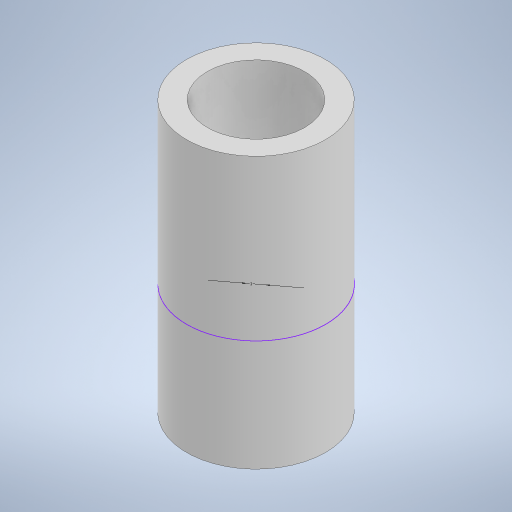
# Autodesk Inventor part: seegoals_adapter_puller_tool_v1
Saved by Autodesk Inventor 2024 (Build 280153000, 153)
## iProperties
Created: 2025-02-17
Part Number: seegoals_adapter_puller_tool_v1
Material: Generic
Document SubType Name: Modeling
Designer: Elev
Density: 1 g/cm^3
Appearance: Default
Author: Elev
Autodesk Inventor part; units mm, degrees
ref_plane "YZ Plane" through (0, 0, 0) normal (1, 0, 0) x (0, 1, 0)
ref_plane "XZ Plane" through (0, 0, 0) normal (0, 1, 0) x (-1, 0, 0)
ref_plane "XY Plane" through (0, 0, 0) normal (0, 0, 1) x (1, 0, 0)
sketch "Sketch1" plane through (0, 0, 0) normal (0, 1, 0) x (-1, 0, 0)
  line L0 (-1.7898, -3.1) -> (-3.5796, 0)
  line L1 (-3.5796, 0) -> (-1.7898, 3.1)
  line L2 (-1.7898, 3.1) -> (1.7898, 3.1)
  line L3 (1.7898, 3.1) -> (3.5796, 0)
  line L4 (3.5796, 0) -> (1.7898, -3.1)
  line L5 (1.7898, -3.1) -> (-1.7898, -3.1)
  circle A0 centre (0, 0) radius 5
  spline S0 degree 2 poles (1.7898, 3.1) (0, 2.8) (-1.7898, 3.1) knots 0 0 0 1 1 1
  spline S1 degree 2 poles (-1.7898, 3.1) (-2.4249, 1.4) (-3.5796, 0) knots 0 0 0 1 1 1
  spline S2 degree 2 poles (-3.5796, 0) (-2.4249, -1.4) (-1.7898, -3.1) knots 0 0 0 1 1 1
  spline S3 degree 2 poles (-1.7898, -3.1) (0, -2.8) (1.7898, -3.1) knots 0 0 0 1 1 1
  spline S4 degree 2 poles (1.7898, -3.1) (2.4249, -1.4) (3.5796, 0) knots 0 0 0 1 1 1
  spline S5 degree 2 poles (3.5796, 0) (2.4249, 1.4) (1.7898, 3.1) knots 0 0 0 1 1 1
  point P0 (0, 0)
  point P1 (0, 0)
  point P2 (0, -3.1)
  point P3 (0, 2.95)
  point P4 (0, 3.1)
  point P5 (-2.5548, 1.475)
  point P6 (-2.5548, -1.475)
  point P7 (0, -2.95)
  point P8 (2.5548, -1.475)
  point P9 (2.5548, 1.475)
  point P10 (1.7898, 3.1)
  point P11 (1.7898, 3.1)
  point P12 (1.7898, 3.1)
  dimension "d0" = 3.1
  dimension "d1" = 10
  dimension "d27" = 0.15
  dimension "d30" = 360
  constraints: 12 end point, 2 midpoint, 1 centre point, 1 coincident, 1 vertical alignment, 56 other
  measures "d0" distance from line of L5 point (0, 0)
  measures "d1" diameter of A0
  measures "d27" distance of point (0, 2.95) point (0, 3.1)
extrude "Extrusion1" add sketch "Sketch1" along normal blind 8 contours S3 L5 | L0 S2 | L1 S1 | S4 L4 | L2 S0 | S5 L3 | A0
sketch "Sketch2" plane through (0, 8, 0) normal (0, 1, 0) x (1, 0, 0)
  circle A0 centre (0, 0) radius 0.5
  circle A1 centre (0, 0) radius 5 projected
  circle A2 centre (0, 0) radius 5
  dimension "d4" = 1
  constraints: 2 centre point, 2 coincident
  measures "d4" diameter of A0
sketch "Sketch5" plane through (0, 0, 0) normal (0, 0, 1) x (1, 0, 0)
  line L0 (5, 8) -> (-5, 8) projected
  line L1 (5, 8) -> (5, 11.5)
  line L2 (5, 11.5) -> (3.5, 11.5)
  line L3 (5, 8) -> (0.5, 8)
  line L4 (0.5, 8) -> (3.5, 11.5)
  line L5 (0, 8) -> (0, 11)
  point P0 (0, 0)
  dimension "d20" = 3.5
  dimension "d21" = 1.5
  dimension "d22" = 4.5
  dimension "d23" = 3
  constraints: 10 end point, 2 vertical, 1 midpoint, 1 perpendicular, 1 point on line
  measures "d20" distance of L0.start L1.end
  measures "d21" distance of L1.end L2.end
  measures "d22" distance of L0.start L3.end
  measures "d23" distance of L5.start L5.end
revolve "Revolution1" add sketch "Sketch5" angle 360 about axis through (0, 8, 0) along (0, 1, 0)
sketch "Sketch7" plane through (0, 11.5, 0) normal (0, 1, 0) x (1, 0, 0)
  circle A0 centre (0, 0) radius 0.5 projected
  circle A1 centre (0, 0) radius 3.5
  circle A2 centre (0, 0) radius 5
  constraints: 2 centre point, 2 coincident
extrude "Extrusion2" add sketch "Sketch7" along normal blind 8 contours A2
body "Solid1"
